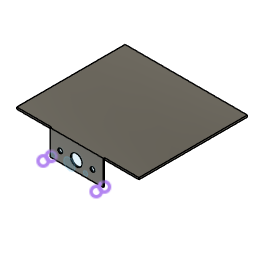
Base (Autodesk Fusion 360 design; units mm, degrees)
Autodesk Fusion 360 part; units mm, degrees
sketch "Sketch1" plane through (0, 0, 0) normal (0, 1, 0) x (1, 0, 0)
  line L0 (0, 0) -> (40.3, 0)
  line L1 (40.3, 0) -> (40.3, 20)
  line L2 (40.3, 20) -> (0, 20)
  line L3 (0, 20) -> (0, 0)
  line L4 (0, 0) -> (0, 5)
  line L5 (0, 20) -> (0, 15)
  line L6 (0, 15) -> (-3.85, 15)
  line L7 (0, 5) -> (-3.85, 5)
  circle A0 centre (-3.85, 15) radius 2.5
  circle A1 centre (-3.85, 5) radius 2.5
  line L8 (40.3, 0) -> (40.3, 5)
  line L9 (40.3, 5) -> (44.15, 5)
  line L10 (40.3, 20) -> (40.3, 15)
  line L11 (40.3, 15) -> (44.15, 15)
  circle A2 centre (44.15, 5) radius 2.5
  circle A3 centre (44.15, 15) radius 2.5
  line L12 (0, 0) -> (-0.5, 0)
  line L13 (-0.5, 0) -> (-0.5, 20)
  line L14 (-0.5, 20) -> (0, 20)
  line L15 (40.3, 20) -> (40.8, 20)
  line L16 (40.8, 20) -> (40.8, 0)
  line L17 (40.8, 0) -> (40.3, 0)
  line L18 (-0.5, 0) -> (-7.5, 0)
  line L19 (-7.5, 0) -> (-7.5, 19.9818)
  line L20 (-7.5, 19.9818) -> (-0.5, 19.9818)
  line L21 (-0.5, 19.9818) -> (-0.5, 0)
  line L22 (40.8, 0) -> (47.8, 0)
  line L23 (47.8, 0) -> (47.8, 20)
  line L24 (47.8, 20) -> (40.8, 20)
  line L25 (40.8, 20) -> (40.8, 0)
  line L26 (-7.5, 19.9818) -> (47.8, 19.9818)
  line L27 (47.8, 19.9818) -> (47.8, 22.9818)
  line L28 (47.8, 22.9818) -> (-7.5, 22.9818)
  line L29 (-7.5, 22.9818) -> (-7.5, 19.9818)
  dimension "d1" = 40.3
  dimension "d2" = 20
  dimension "d3" = 5
  dimension "d4" = 5
  dimension "d5" = 3.85
  dimension "d6" = 3.85
  dimension "d7" = 5
  dimension "d8" = 5
  dimension "d9" = 5
  dimension "d10" = 3.85
  dimension "d11" = 5
  dimension "d12" = 3.85
  dimension "d13" = 5
  dimension "d14" = 5
  dimension "d15" = 0.5
  dimension "d16" = 7
  dimension "d17" = 7
  dimension "d18" = 3
  constraint horizontal L0
  constraint vertical L1
  constraint horizontal L2
  constraint vertical L3
  constraint coincident L0.start L3.end
  constraint perpendicular L0 L4
  constraint perpendicular L2 L5
  constraint perpendicular L3 L6
  constraint perpendicular L4 L7
  constraint coincident L6.end A0.centre
  constraint coincident L7.end A1.centre
  constraint perpendicular L0 L8
  constraint perpendicular L1 L9
  constraint perpendicular L2 L10
  constraint perpendicular L1 L11
  constraint coincident L9.end A2.centre
  constraint coincident L11.end A3.centre
  constraint perpendicular L3 L12
  constraint perpendicular L6 L13
  constraint perpendicular L1 L15
  constraint perpendicular L11 L16
  constraint perpendicular L1 L17
  constraint horizontal L18
  constraint vertical L19
  constraint horizontal L20
  constraint vertical L21
  constraint horizontal L22
  constraint vertical L23
  constraint horizontal L24
  constraint vertical L25
  constraint horizontal L26
  constraint vertical L27
  constraint horizontal L28
  constraint vertical L29
  measures "d1" distance of L0.start L0.end
  measures "d2" distance of L0.start L2.end
  measures "d3" distance of L0.start L4.end
  measures "d4" distance of L2.end L5.end
  measures "d5" distance of L5.end L6.end
  measures "d6" distance of L4.end L7.end
  measures "d7" diameter of A0
  measures "d8" diameter of A1
  measures "d9" distance of L0.end L8.end
  measures "d10" distance of L8.end L9.end
  measures "d11" distance of L1.end L10.end
  measures "d12" distance of L10.end L11.end
  measures "d13" diameter of A2
  measures "d14" diameter of A3
  measures "d15" distance of L1.end L15.end
  measures "d16" distance of L12.end L18.end
  measures "d17" distance of L16.end L22.end
  measures "d18" distance of L19.end L28.end
extrude "Extrude1" add sketch "Sketch1" along normal blind 8.5 contours L13 L18 L19 L20 L21 L26 | L16 L22 L23 L25 L26 | L2 L13 L14 L15 L20 L24 L26 L27 L28 L29 makes body 1 at (29.3667, 2.8333, -22.9818) makes body 2 at (40.8, 2.8333, -13.3212)
sketch "Sketch2" plane through (0, 0, -22.9818) normal (0, 0, -1) x (1, 0, 0)
  line L0 (47.8, 0) -> (-7.5, 0)
  line L1 (-7.5, 0) -> (-7.5, -8.5)
  line L2 (-7.5, -8.5) -> (47.8, -8.5)
  line L3 (47.8, -8.5) -> (47.8, 0)
  line L4 (20.15, 0) -> (18.65, 0)
  line L5 (18.65, 0) -> (18.65, -8.5)
  line L6 (18.65, -8.5) -> (20.15, -8.5)
  line L7 (20.15, -8.5) -> (20.15, 0)
  line L8 (20.15, -8.5) -> (21.65, -8.5)
  line L9 (21.65, -8.5) -> (21.65, 0)
  line L10 (21.65, 0) -> (20.15, 0)
  line L11 (20.15, 0) -> (20.15, -8.5)
  dimension "d21" = 1.5
  dimension "d22" = 1.5
  constraint horizontal L4
  constraint vertical L5
  constraint horizontal L6
  constraint vertical L7
  constraint midpoint L0 L4.start
  constraint horizontal L8
  constraint vertical L9
  constraint horizontal L10
  constraint vertical L11
  measures "d21" distance of L4.start L4.end
  measures "d22" distance of L6.end L8.end
extrude "Extrude2" add sketch "Sketch2" along normal blind 17 contours L0 L2 L7 L8 L9 L10 L11 | L0 L2 L4 L5 L6 L7 L11 bodies 1
extrude "Extrude3" add 1 faces at (21.65, 5.6667, -34.3151) along direction (1, 0, 0) blind 10 on bodies 1 bodies 1
extrude "Extrude4" add 1 faces at (18.65, 2.8333, -34.3151) along direction (-1, 0, 0) blind 10 on bodies 1 bodies 1
sketch "Sketch3" plane through (0, 8.5, 0) normal (0, 1, 0) x (-1, 0, 0)
  circle A0 centre (3.85, -5) radius 2.5
  circle A1 centre (3.85, -15) radius 2.5
  line L0 (-47.8, -20) -> (-47.8, -22.9818)
  line L1 (-47.8, -22.9818) -> (-31.65, -22.9818)
  line L2 (-31.65, -22.9818) -> (-31.65, -39.9818)
  line L3 (-31.65, -39.9818) -> (-8.65, -39.9818)
  line L4 (-8.65, -39.9818) -> (-8.65, -22.9818)
  line L5 (-8.65, -22.9818) -> (7.5, -22.9818)
  line L6 (7.5, -22.9818) -> (7.5, 0)
  line L7 (7.5, 0) -> (0.5, 0)
  line L8 (0.5, 0) -> (0.5, -20)
  line L9 (0.5, -20) -> (0, -20)
  line L10 (0, -20) -> (-47.8, -20)
  line L11 (0.5, -20) -> (7.5, -20)
  constraint coincident L8.end L9.start
  constraint coincident L6 L11.end
  constraint perpendicular L6 L11
sketch "Sketch5" plane through (0, 0, 0) normal (0, -1, 0) x (1, 0, 0)
extrude "Extrude5" cut sketch "Sketch3" against normal blind 5 contours L6 L7 L8 L11 bodies 1
extrude "Extrude6" cut 1 faces at (44.3123, 8.5, -0.8357) along direction (0, -1, 0) blind 5 on bodies 2 bodies 2
extrude "Extrude7" add 1 faces at (16.3167, 2.8333, -39.9818) along direction (0, 0, -1) blind 7 on bodies 1 bodies 1
extrude "Extrude8" cut 1 faces at (23.9833, 8.5, -30.9818) along direction (0, -1, 0) blind 5 on bodies 1 bodies 1
sketch "Sketch7" plane through (0, 3.5, 0) normal (0, 1, 0) x (-1, 0, 0)
  circle A0 centre (3.85, -5) radius 2.5
  circle A1 centre (3.85, -15) radius 2.5
  line L0 (7.5, -22.9818) -> (7.5, 0)
  line L1 (7.5, 0) -> (0.5, 0)
  line L2 (0.5, 0) -> (0.5, -20)
  line L3 (0.5, -20) -> (0, -20)
  line L4 (0, -20) -> (-47.8, -20)
  line L5 (-47.8, -20) -> (-47.8, -22.9818)
  line L6 (-47.8, -22.9818) -> (-31.65, -22.9818)
  line L7 (-31.65, -22.9818) -> (-31.65, -46.9818)
  line L8 (-31.65, -46.9818) -> (-8.65, -46.9818)
  line L9 (-8.65, -46.9818) -> (-8.65, -22.9818)
  line L10 (-8.65, -22.9818) -> (7.5, -22.9818)
  circle A2 centre (-20, -37.5) radius 2.5
  circle A3 centre (-27, -37.5) radius 1
  circle A4 centre (-13, -37.5) radius 1
  circle A5 centre (-20, -44.5) radius 1
  circle A6 centre (-20, -30.5) radius 1
  dimension "d37" = 5
  dimension "d38" = 2
  dimension "d39" = 2
  dimension "d40" = 2
  dimension "d41" = 2
  measures "d37" diameter of A2
  measures "d38" diameter of A3
  measures "d39" diameter of A4
  measures "d40" diameter of A5
  measures "d41" diameter of A6
hole "Hole1" at (19.9998, 3.5, -37.5) direction (0, -1, 0) diameter 5 depth 4 tip angle 118 bodies 1
hole "Hole2" at (20, 3.5, -30.5002) direction (0, -1, 0) diameter 2 depth 4 tip angle 118 bodies 1
hole "Hole3" at (13, 3.5, -37.5) at (20, 3.5, -44.5) at (27, 3.5, -37.5) direction (0, -1, 0) diameter 2 depth 4 tip angle 118 bodies 1
move_body "Move1" bodies 1 to x (1, 0, 0) y (0, 1, 0) z (0, 0, 1) at (-20.0882, -24.3535, -4.2653)
delete_face "DeleteFace1" 1 faces at (-20.5882, -23.1868, -10.932) on bodies 1
delete_face "DeleteFace2" 1 faces at (-22.5882, -23.1868, -24.2653) on bodies 1
delete_face "DeleteFace3" 1 faces at (-0.8041, -22.0202, -35.4637) on bodies 1
delete_face "DeleteFace4" 1 faces at (-0.8041, -22.0202, -49.4635) on bodies 1
extrude "Extrude9" cut 1 faces at (-3.7715, -23.1868, -51.2471) along direction (0, 0, 1) blind 5 on bodies 1 bodies 1
sketch "Sketch8" plane through (0, -24.3535, 0) normal (0, -1, 0) x (1, 0, 0)
  line L0 (-11.4382, -46.2471) -> (11.5618, -46.2471)
  circle A0 centre (-0.0884, -41.7653) radius 2.5
  circle A1 centre (6.9118, -41.7653) radius 1
  circle A2 centre (-7.0882, -41.7653) radius 1
sketch "Sketch9" plane through (0, -20.8535, 0) normal (0, 1, 0) x (-1, 0, 0)
  circle A0 centre (0.0884, -41.7653) radius 2.5
  circle A1 centre (-6.9118, -41.7653) radius 1
  circle A2 centre (7.0882, -41.7653) radius 1
  line L0 (-11.5618, -46.2471) -> (11.4382, -46.2471)
sketch "Sketch10" plane through (0, 0, -24.2653) normal (0, 0, 1) x (-1, 0, 0)
delete_face "DeleteFace5" 1 faces at (-27.5882, -23.1868, -26.2532) on bodies 1
delete_face "DeleteFace6" 2 faces at (27.7118, -23.1868, -25.2592) (22.3285, -23.1868, -27.2471) on bodies 1
sketch "Sketch11" plane through (0, -24.3535, 0) normal (0, -1, 0) x (1, 0, 0)
  line L0 (-11.4382, -46.2471) -> (11.5618, -46.2471)
  circle A0 centre (-0.0884, -41.7653) radius 2.5
  circle A1 centre (6.9118, -41.7653) radius 1
  circle A2 centre (-7.0882, -41.7653) radius 1
sketch "Sketch12" plane through (0, 0, -24.2653) normal (0, 0, 1) x (-1, 0, 0)
sketch "Sketch13" plane through (0, -20.8535, 0) normal (0, 1, 0) x (-1, 0, 0)
  line L0 (-11.5618, -46.2471) -> (11.4382, -46.2471)
  circle A0 centre (0.0884, -41.7653) radius 2.5
  circle A1 centre (-6.9118, -41.7653) radius 1
  circle A2 centre (7.0882, -41.7653) radius 1
delete_face "DeleteFace7" 2 faces at (-16.8215, -23.1868, -27.2471) (-27.5882, -23.1868, -26.2532) on bodies 1
delete_face "DeleteFace8" 1 faces at (46.6376, 1.1667, -15.2489) on bodies 2
delete_face "DeleteFace9" 1 faces at (46.6469, 2.3333, -4.8754) on bodies 2
delete_face "DeleteFace10" 6 faces at (43.1333, 0, -6.6606) (43.1333, 1.1667, 0) (47.8, 1.1667, -6.6606) (43.1333, 3.5, -6.6606) (40.8, 1.1667, -13.3212) (43.1333, 1.1667, -19.9818) on bodies 2
extrude "Extrude10" cut 1 faces at (3.8951, -23.1868, -24.2653) along direction (0, 0, -1) blind 13 on bodies 1 bodies 1
extrude "Extrude11" add 1 faces at (3.8951, -23.1868, -37.2653) along direction (0, 0, 1) blind 2 on bodies 1 bodies 1
sketch "Sketch14" plane through (0, -20.8535, 0) normal (0, 1, 0) x (-1, 0, 0)
  line L0 (-11.5618, -35.2653) -> (-11.5618, -46.2471)
  line L1 (-11.5618, -46.2471) -> (11.4382, -46.2471)
  line L2 (11.4382, -46.2471) -> (11.4382, -35.2653)
  line L3 (11.4382, -35.2653) -> (-11.5618, -35.2653)
  circle A0 centre (0.0884, -41.7653) radius 2.5
  circle A1 centre (-6.9118, -41.7653) radius 1
  circle A2 centre (7.0882, -41.7653) radius 1
  line L4 (-11.5618, -37.046) -> (11.4382, -37.046)
  constraint coincident L0 L4.start
  constraint coincident L2 L4.end
  constraint perpendicular L2 L4
extrude "Extrude12" add sketch "Sketch14" along normal blind 20 contours L0 L2 L3 L4 bodies 1
sketch "Sketch15" plane through (-11.4382, 0, 0) normal (-1, 0, 0) x (0, -1, 0)
  line L0 (20.8535, -37.046) -> (20.8535, -46.2471)
  line L1 (20.8535, -46.2471) -> (24.3535, -46.2471)
  line L2 (24.3535, -46.2471) -> (24.3535, -35.2653)
  line L3 (24.3535, -35.2653) -> (0.8535, -35.2653)
  line L4 (0.8535, -35.2653) -> (0.8535, -37.046)
  line L5 (0.8535, -37.046) -> (20.8535, -37.046)
  line L6 (20.8535, -37.046) -> (20.8535, -35.2653)
  constraint coincident L0.start L5.end
  constraint perpendicular L3 L6
extrude "Extrude13" add sketch "Sketch15" along normal blind 5 contours L3 L4 L5 L6 bodies 1
sketch "Sketch16" plane through (11.5618, 0, 0) normal (1, 0, 0) x (0, 1, 0)
  line L0 (-24.3535, -35.2653) -> (-24.3535, -46.2471)
  line L1 (-24.3535, -46.2471) -> (-20.8535, -46.2471)
  line L2 (-20.8535, -46.2471) -> (-20.8535, -37.046)
  line L3 (-20.8535, -37.046) -> (-0.8535, -37.046)
  line L4 (-0.8535, -37.046) -> (-0.8535, -35.2653)
  line L5 (-0.8535, -35.2653) -> (-24.3535, -35.2653)
  line L6 (-20.8535, -37.046) -> (-20.8535, -35.2653)
  constraint coincident L2.end L3.start
  constraint coincident L5 L6.end
  constraint perpendicular L5 L6
extrude "Extrude14" add sketch "Sketch16" along normal blind 5 contours L3 L4 L5 L6 bodies 1
extrude "Extrude15" cut 1 faces at (0.0117, -24.3535, -36.5986) along direction (0, 1, 0) blind 3 on bodies 1 bodies 1
sketch "Sketch17" plane through (0, 0, -37.046) normal (0, 0, -1) x (1, 0, 0)
  line L0 (11.5618, 20.8535) -> (-11.4382, 20.8535)
  line L1 (-11.4382, 20.8535) -> (-16.4382, 20.8535)
  line L2 (-16.4382, 20.8535) -> (-16.4382, 0.8535)
  line L3 (-16.4382, 0.8535) -> (16.5618, 0.8535)
  line L4 (16.5618, 0.8535) -> (16.5618, 20.8535)
  line L5 (16.5618, 20.8535) -> (11.5618, 20.8535)
extrude "Extrude16" cut sketch "Sketch17" against normal blind 1 bodies 1
sketch "Sketch18" plane through (0, -0.8535, 0) normal (0, 1, 0) x (-1, 0, 0)
  line L0 (-16.5618, -36.046) -> (16.4382, -36.046)
  line L1 (16.4382, -36.046) -> (16.4382, -35.2653)
  line L2 (16.4382, -35.2653) -> (-16.5618, -35.2653)
  line L3 (-16.5618, -35.2653) -> (-16.5618, -36.046)
extrude "Extrude17" add sketch "Sketch18" along normal blind 27 bodies 1
sketch "Sketch19" plane through (-16.4382, 0, 0) normal (-1, 0, 0) x (0, -1, 0)
  line L0 (-26.1465, -36.046) -> (20.8535, -36.046)
  line L1 (20.8535, -36.046) -> (20.8535, -35.2653)
  line L2 (20.8535, -35.2653) -> (-26.1465, -35.2653)
  line L3 (-26.1465, -35.2653) -> (-26.1465, -36.046)
extrude "Extrude18" add sketch "Sketch19" along normal blind 10 bodies 1
extrude "Extrude19" add 1 faces at (16.5618, -5.1868, -35.5255) along direction (1, 0, 0) blind 10 on bodies 1 bodies 1
equation "d5 = ( ( 48 - 40.3 ) / 2 ) * 1 mm"
